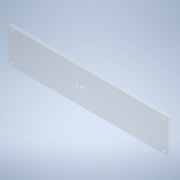
# Autodesk Inventor part: Template-Fixture-Bottom
Saved by Autodesk Inventor 2021 (Build 250183000, 183)
## iProperties
Created: 2020-06-16
Part Number: Template-Fixture-Bottom
Material: Polycarbonate, Clear
Document SubType Name: Modeling
Designer: lucas
Density: 1.2 g/cm^3
Appearance: Polycarbonate - Clear
Project: 4Wire-FDM
Author: lucas
Revision Number: RLS_004
Autodesk Inventor part; units mm, degrees
ref_plane "YZ Plane" through (0, 0, 0) normal (1, 0, 0) x (0, 1, 0)
ref_plane "XZ Plane" through (0, 0, 0) normal (0, 1, 0) x (-1, 0, 0)
ref_plane "XY Plane" through (0, 0, 0) normal (0, 0, 1) x (1, 0, 0)
sketch "Sketch1" plane through (0, 0, 0) normal (0, 0, 1) x (1, 0, 0)
  line L0 (93.3916, -12.6) -> (93.3916, 12.6)
  line L1 (53.9763, -12.6) -> (93.3916, -12.6)
  line L2 (53.9763, -15.2) -> (53.9763, -12.6)
  line L3 (38.2753, -15.2) -> (53.9763, -15.2)
  line L4 (38.2753, -15.2) -> (23.4296, -15.2)
  line L5 (23.4296, -12.6) -> (23.4296, -15.2)
  line L6 (-76.0546, -12.6) -> (23.4296, -12.6)
  line L7 (23.4296, 12.6) -> (-76.0546, 12.6)
  line L8 (23.4296, 15.2) -> (23.4296, 12.6)
  line L9 (-76.0546, 12.6) -> (-76.0546, -12.6)
  line L10 (-70.1, 10) -> (-66.9, 10)
  line L11 (-66.9, -10) -> (-70.1, -10)
  line L12 (23.4296, 15.2) -> (53.9763, 15.2)
  line L13 (53.9763, 15.2) -> (53.9763, 12.6)
  line L14 (53.9763, 12.6) -> (93.3916, 12.6)
  line L15 (-77.0546, 13.6) -> (22.4296, 13.6)
  line L16 (22.4296, 13.6) -> (22.4296, 16.2)
  line L17 (22.4296, 16.2) -> (54.9763, 16.2)
  line L18 (54.9763, 16.2) -> (54.9763, 13.6)
  line L19 (54.9763, 13.6) -> (94.3916, 13.6)
  line L20 (94.3916, 13.6) -> (94.3916, -13.6)
  line L21 (94.3916, -13.6) -> (54.9763, -13.6)
  line L22 (54.9763, -13.6) -> (54.9763, -16.2)
  line L23 (54.9763, -16.2) -> (38.2753, -16.2)
  line L24 (38.2753, -16.2) -> (22.4296, -16.2)
  line L25 (22.4296, -16.2) -> (22.4296, -13.6)
  line L26 (22.4296, -13.6) -> (-77.0546, -13.6)
  line L27 (-77.0546, -13.6) -> (-77.0546, 13.6)
  line L28 (22.4296, -16.2) -> (22.4296, -20.2) construction
  line L29 (22.4296, -20.2) -> (-87.5704, -20.2)
  line L30 (-87.5704, -20.2) -> (-87.5704, 20.2)
  line L31 (-87.5704, 20.2) -> (22.4296, 20.2)
  line L32 (104.4296, -20.2) -> (22.4296, -20.2)
  line L33 (22.4296, 20.2) -> (104.4296, 20.2)
  line L34 (104.4296, 20.2) -> (104.4296, -20.2)
  circle A0 centre (-82.5704, 17.2) radius 1.6
  circle A1 centre (-82.5704, -17.2) radius 1.6
  circle A2 centre (99.4296, 17.2) radius 1.6
  circle A3 centre (99.4296, -17.2) radius 1.6
  dimension "d0" = 1
  dimension "d1" = 4
  dimension "d2" = 110
  dimension "d3" = 40.4
  dimension "d5" = 82
  dimension "d18" = 5
  dimension "d19" = 5
  dimension "d20" = 3
  dimension "d21" = 3
  dimension "d22" = 5
  dimension "d23" = 3
  dimension "d24" = 5
  dimension "d25" = 3
  constraints: 70 end point, 7 perpendicular, 4 centre point, 2 horizontal, 1 parallel, 1 point on line, 1 vertical, 12 other
  measures "d0" distance between parallel lines of L7 L15
  measures "d1" distance of L24.end L28.end
  measures "d2" distance of L28.end L29.end
  measures "d3" distance of L29.end L30.end
  measures "d5" distance of L31.end L33.end
  measures "d18" distance from line of L30 A0.centre
  measures "d19" distance from line of L30 A1.centre
  measures "d20" distance from line of L29 A1.centre
  measures "d21" distance from line of L31 A0.centre
  measures "d22" distance from line of L34 A3.centre
  measures "d23" distance from line of L32 A3.centre
  measures "d24" distance from line of L34 A2.centre
  measures "d25" distance from line of L33 A2.centre
extrude "Extrusion1" add sketch "Sketch1" against normal blind 4 contours L1 L2 L3 L4 L5 L6 L9 L7 L8 L12 L13 L14 L0 | L15 L16 L17 L18 L19 L20 L21 L22 L23 L24 L25 L26 L27 | L29 L30 L31 L33 L34 L32
sketch "Sketch3" plane through (0, 0, 0) normal (0, 0, 1) x (1, 0, 0)
  arc A0 (-9.9934, 7) -> (-9.9934, -7) centre (-9.9934, 0) ccw projected
  line L0 (21.0066, 7) -> (-9.9934, 7) projected
  line L1 (-9.9934, -7) -> (21.0066, -7) projected
  arc A1 (21.0066, -7) -> (21.0066, 7) centre (21.0066, 0) ccw projected
  circle A2 centre (0, 0) radius 2
  line L2 (0, 0) -> (5, 0) construction
  line L3 (0, 0) -> (-5, 0)
  line L4 (-5, 3) -> (-5, -3) construction
  line L5 (-5.5, 3) -> (-5.5, -3)
  line L6 (-4.5, -3) -> (-4.5, 3)
  arc A3 (-4.5, 3) -> (-5.5, 3) centre (-5, 3) ccw
  arc A4 (-5.5, -3) -> (-4.5, -3) centre (-5, -3) ccw
  line L7 (5, 3) -> (5, -3) construction
  line L8 (4.5, 3) -> (4.5, -3)
  line L9 (5.5, -3) -> (5.5, 3)
  arc A5 (5.5, 3) -> (4.5, 3) centre (5, 3) ccw
  arc A6 (4.5, -3) -> (5.5, -3) centre (5, -3) ccw
  dimension "d26" = 4
  dimension "d27" = 5
  dimension "d28" = 5
  dimension "d29" = 3
  dimension "d30" = 1
  dimension "d31" = 3
  dimension "d32" = 1
  constraints: 20 end point, 8 point on circle, 8 tangent, 5 centre point, 3 parallel, 2 horizontal, 2 midpoint, 1 coincident, 1 vertical
  measures "d26" diameter of A2
  measures "d27" distance of L2.start L2.end
  measures "d28" distance of L2.start L3.end
  measures "d29" distance of L3.end L4.end
  measures "d30" diameter of A4
  measures "d31" distance of L2.end L7.end
  measures "d32" diameter of A6
extrude "Extrusion3" cut sketch "Sketch3" against normal through all contours A2 | L6 A4 L5 A3 | A5 L9 A6 L8
body "Solid1"
